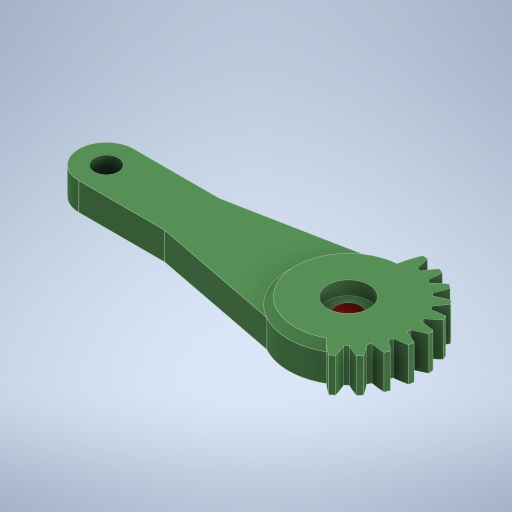
# Autodesk Inventor part: mechanism_1L
Saved by Autodesk Inventor 2023 (Build 270158000, 158)
## iProperties
Created: 2024-07-18
Part Number: mechanism_1L
Material: Generic
Document SubType Name: Modeling
Designer: Swoby
Density: 1 g/cm^3
Appearance: Default
Author: Swoby
Autodesk Inventor part; units mm, degrees
ref_plane "YZ Plane" through (0, 0, 0) normal (1, 0, 0) x (0, 1, 0)
ref_plane "XZ Plane" through (0, 0, 0) normal (0, 1, 0) x (-1, 0, 0)
ref_plane "XY Plane" through (0, 0, 0) normal (0, 0, 1) x (1, 0, 0)
sketch "Sketch1" plane through (0, 0, 0) normal (0, 1, 0) x (-1, 0, 0)
  circle A0 centre (0, 0) radius 1.75
  circle A1 centre (-35.232, 0) radius 1.75
  line L0 (0, 0) -> (-35.232, 0)
  line L1 (4, 0) -> (-39.232, 0) construction
  line L2 (0, -4) -> (-35.232, -4)
  line L3 (-35.232, 4) -> (-27.492, 4)
  arc A2 (0, -4) -> (0, 4) centre (0, 0) ccw
  arc A3 (-35.232, 4) -> (-35.232, -4) centre (-35.232, 0) ccw
  arc A4 (-26.5195, 0) -> (-27.492, 4) centre (-35.232, 0) ccw construction
  line L4 (-27.492, 4) -> (0, 4)
  arc A5 (-27.492, -4) -> (-26.5195, 0) centre (-35.232, 0) ccw construction
  arc A6 (-27.492, 4) -> (-27.492, -4) centre (-35.232, 0) ccw
  point P0 (-17.616, 0)
  dimension "d0" = 35.232
  dimension "d1" = 3.5
  dimension "d2" = 3.5
  dimension "d3" = 4
  dimension "d6" = 17.425
  constraints: 12 end point, 12 point on circle, 7 centre point, 6 tangent, 4 coincident, 4 point on line, 2 horizontal, 2 parallel, 1 midpoint
  measures "d0" distance of L0.end point (0, 0)
  measures "d1" diameter of A0
  measures "d2" diameter of A1
  measures "d3" radius of A2
  measures "d6" diameter of A4
extrude "Extrusion1" add sketch "Sketch1" along normal blind 4
sketch "Sketch2" plane through (0, 0, 0) normal (0, -1, 0) x (1, 0, 0)
  line L0 (27.492, -4) -> (0, -4) projected
  arc A0 (27.492, -4) -> (27.492, 4) centre (35.232, 0) ccw projected
  line L1 (0, 4) -> (27.492, 4) projected
  arc A1 (0, 4) -> (0, -4) centre (0, 0) ccw projected
  circle A2 centre (35.232, 0) radius 1.75 projected
  circle A3 centre (0, 0) radius 1.75 projected
  circle A4 centre (35.232, 0) radius 1.75 projected
  line L2 (35.232, 0) -> (35.232, -9.5201)
  line L3 (35.232, 0) -> (40.5265, 9.1703)
  arc A5 (35.232, -10.589) -> (40.5265, 9.1703) centre (35.232, 0) ccw
  line L4 (35.2321, 0.0005) -> (35.2321, 10.589) construction
  line L5 (35.2321, 0.0005) -> (40.5265, -9.1694) construction
  arc A6 (40.5265, -9.1694) -> (35.4759, -10.5852) centre (35.2321, 0.0005) ccw construction
  line L6 (35.2321, 0.0005) -> (42.6249, -4.6093) construction
  line L7 (35.2321, 0.0005) -> (42.7778, -4.3544) construction
  line L8 (35.2321, 0.0005) -> (42.4633, -4.8588) construction
  line L9 (35.2321, 0.0005) -> (43.506, -2.7279) construction
  line L10 (35.2321, 0.0005) -> (45.0385, -3.9936) construction
  line L11 (35.2321, 0.0005) -> (44.7425, -4.6546) construction
  arc A7 (45.0385, -3.9936) -> (43.506, -2.7279) centre (34.8965, -14.7131) ccw
  arc A8 (42.7778, -4.3544) -> (44.7425, -4.6546) centre (45.9843, 10.05) ccw
  arc A9 (44.7425, -4.6546) -> (45.0385, -3.9936) centre (35.2321, 0.0005) ccw
  arc A10 (42.4633, -4.8588) -> (42.7778, -4.3544) centre (35.2321, 0.0005) ccw
  line L12 (35.2321, 0.0005) -> (43.9353, -0.3948) construction
  line L13 (35.2321, 0.0005) -> (43.6728, -2.1574) construction
  line L14 (35.2321, 0.0005) -> (45.7524, -1.2001) construction
  line L15 (35.2321, 0.0005) -> (45.6457, -1.9165) construction
  arc A11 (43.6728, -2.1574) -> (43.9353, -0.3948) centre (35.2323, 0.0004) ccw construction
  arc A12 (43.506, -2.7279) -> (43.6728, -2.1574) centre (35.2323, 0.0004) ccw
  arc A13 (45.6457, -1.9165) -> (45.7524, -1.2001) centre (35.2321, 0.0005) ccw
  arc A14 (45.7524, -1.2001) -> (45.7767, 0.9637) centre (35.2321, 0.0005) ccw construction
  arc A15 (43.6728, -2.1574) -> (45.6457, -1.9165) centre (42.8748, 12.578) ccw
  arc A16 (45.7524, -1.2001) -> (43.9353, -0.3948) centre (38.8781, -14.2582) ccw
  line L16 (35.2321, 0.0005) -> (43.942, 0.1996) construction
  line L17 (35.2321, 0.0005) -> (45.7767, 0.9637) construction
  line L18 (35.2321, 0.0005) -> (45.6862, 1.6823) construction
  line L19 (35.2321, 0.0005) -> (43.7193, 1.9676) construction
  arc A17 (45.7767, 0.9637) -> (45.6862, 1.6823) centre (35.2321, 0.0005) ccw
  arc A18 (45.6862, 1.6823) -> (45.126, 3.7725) centre (35.2321, 0.0005) ccw construction
  arc A19 (43.942, 0.1996) -> (43.7193, 1.9676) centre (35.2323, 0.0004) ccw construction
  arc A20 (43.9353, -0.3948) -> (43.942, 0.1996) centre (35.2323, 0.0004) ccw
  arc A21 (43.7193, 1.9676) -> (43.5654, 2.5417) centre (35.2323, 0.0004) ccw
  arc A22 (43.942, 0.1996) -> (45.7767, 0.9637) centre (39.1986, 14.1734) ccw
  arc A23 (45.6862, 1.6823) -> (43.7193, 1.9676) centre (42.5894, -12.7461) ccw
  line L20 (35.2321, 0.0005) -> (43.5654, 2.5417) construction
  line L21 (35.2321, 0.0005) -> (45.126, 3.7725) construction
  line L22 (35.2321, 0.0005) -> (44.845, 4.4401) construction
  line L23 (35.2321, 0.0005) -> (42.874, 4.1841) construction
  line L24 (35.2321, 0.0005) -> (42.5709, 4.6955) construction
  line L25 (35.2321, 0.0005) -> (43.7417, 6.3016) construction
  line L26 (35.2321, 0.0005) -> (43.291, 6.8686) construction
  line L27 (35.2321, 0.0005) -> (41.4621, 6.0905) construction
  arc A24 (43.5654, 2.5417) -> (42.874, 4.1841) centre (35.2323, 0.0004) ccw construction
  arc A25 (42.5709, 4.6955) -> (41.4621, 6.0905) centre (35.2323, 0.0004) ccw construction
  arc A26 (42.874, 4.1841) -> (42.5709, 4.6955) centre (35.2323, 0.0004) ccw
  arc A27 (41.4621, 6.0905) -> (41.0323, 6.5011) centre (35.2323, 0.0004) ccw
  arc A28 (43.7417, 6.3016) -> (43.291, 6.8686) centre (35.2321, 0.0005) ccw
  arc A29 (43.291, 6.8686) -> (41.7264, 8.3636) centre (35.2321, 0.0005) ccw construction
  arc A30 (44.845, 4.4401) -> (43.7417, 6.3016) centre (35.2321, 0.0005) ccw construction
  arc A31 (45.126, 3.7725) -> (44.845, 4.4401) centre (35.2321, 0.0005) ccw
  arc A32 (43.291, 6.8686) -> (41.4621, 6.0905) centre (48.1409, -7.0686) ccw
  arc A33 (42.5709, 4.6955) -> (43.7417, 6.3016) centre (31.2583, 14.1714) ccw
  arc A34 (44.845, 4.4401) -> (42.874, 4.1841) centre (45.7553, -10.2888) ccw
  arc A35 (43.5654, 2.5417) -> (45.126, 3.7725) centre (35.2283, 14.718) ccw
  line L28 (35.2321, 0.0005) -> (41.0323, 6.5011) construction
  line L29 (35.2321, 0.0005) -> (41.7264, 8.3636) construction
  line L30 (35.2321, 0.0005) -> (41.1395, 8.788) construction
  line L31 (35.2321, 0.0005) -> (39.5882, 7.5452) construction
  arc A36 (41.7264, 8.3636) -> (41.1395, 8.788) centre (35.2321, 0.0005) ccw
  arc A37 (41.1395, 8.788) -> (35.2321, 10.589) centre (35.2321, 0.0005) ccw construction
  arc A38 (41.1395, 8.788) -> (39.5882, 7.5452) centre (49.5694, -3.3242) ccw
  arc A39 (41.0323, 6.5011) -> (41.7264, 8.3636) centre (27.5829, 12.5742) ccw
  line L32 (35.2321, 0.0005) -> (43.5975, -6.4908) construction
  line L33 (35.2321, 0.0005) -> (43.1341, -7.0475) construction
  line L34 (35.2321, 0.0005) -> (41.3233, -6.2284) construction
  line L35 (35.2321, 0.0005) -> (40.8844, -6.6293) construction
  line L36 (35.2321, 0.0005) -> (41.5362, -8.5068) construction
  line L37 (35.2321, 0.0005) -> (40.9399, -8.9179) construction
  line L38 (35.2321, 0.0005) -> (39.4172, -7.6407) construction
  line L39 (35.2321, 0.0005) -> (38.8864, -7.9082) construction
  line L40 (35.2321, 0.0005) -> (39.0076, -9.892) construction
  line L41 (35.2321, 0.0005) -> (38.3225, -10.127) construction
  line L42 (35.2321, 0.0005) -> (37.2007, -8.4863) construction
  line L43 (35.2321, 0.0005) -> (36.6174, -8.6008) construction
  line L44 (35.2321, 0.0005) -> (36.199, -10.5438) construction
  line L45 (35.2321, 0.0005) -> (35.4759, -10.5852) construction
  line L46 (35.2321, 0.0005) -> (34.8383, -8.7031) construction
  arc A40 (43.5975, -6.4908) -> (42.4633, -4.8588) centre (30.9397, -14.0771) ccw
  arc A41 (43.5975, -6.4908) -> (45.6457, -1.9165) centre (35.2321, 0.0005) ccw construction
  arc A42 (43.1341, -7.0475) -> (43.5975, -6.4908) centre (35.2321, 0.0005) ccw
  arc A43 (41.3233, -6.2284) -> (43.506, -2.7279) centre (35.2323, 0.0004) ccw construction
  arc A44 (40.8844, -6.6293) -> (41.3233, -6.2284) centre (35.2323, 0.0004) ccw
  arc A45 (40.9399, -8.9179) -> (41.5362, -8.5068) centre (35.2321, 0.0005) ccw
  arc A46 (41.5362, -8.5068) -> (43.1341, -7.0475) centre (35.2321, 0.0005) ccw construction
  arc A47 (38.3225, -10.127) -> (39.0076, -9.892) centre (35.2321, 0.0005) ccw
  arc A48 (39.0076, -9.892) -> (40.9399, -8.9179) centre (35.2321, 0.0005) ccw construction
  arc A49 (35.4759, -10.5852) -> (36.199, -10.5438) centre (35.2321, 0.0005) ccw
  arc A50 (36.199, -10.5438) -> (38.3225, -10.127) centre (35.2321, 0.0005) ccw construction
  arc A51 (38.8864, -7.9082) -> (39.4172, -7.6407) centre (35.2323, 0.0004) ccw
  arc A52 (39.4172, -7.6407) -> (40.8844, -6.6293) centre (35.2323, 0.0004) ccw construction
  arc A53 (37.2007, -8.4863) -> (38.8864, -7.9082) centre (35.2323, 0.0004) ccw construction
  arc A54 (36.6174, -8.6008) -> (37.2007, -8.4863) centre (35.2323, 0.0004) ccw
  arc A55 (41.3233, -6.2284) -> (43.1341, -7.0475) centre (48.2967, 6.777) ccw
  arc A56 (41.5362, -8.5068) -> (40.8844, -6.6293) centre (27.3013, -12.3973) ccw
  arc A57 (39.4172, -7.6407) -> (40.9399, -8.9179) centre (49.6404, 3.0014) ccw
  arc A58 (39.0076, -9.892) -> (38.8864, -7.9082) centre (24.2509, -9.7983) ccw
  arc A59 (37.2007, -8.4863) -> (38.3225, -10.127) centre (49.9158, -0.9967) ccw
  arc A60 (36.199, -10.5438) -> (36.6174, -8.6008) centre (22.0147, -6.4728) ccw
  arc A61 (34.8383, -8.7031) -> (35.4759, -10.5852) centre (49.1022, -4.92) ccw
  point P0 (37.8164, 8.3636)
  point P1 (39.5883, 7.5452)
  point P2 (42.7783, -4.3545)
  point P3 (42.4636, -4.8592)
  point P4 (41.3238, -6.2287)
  point P5 (40.8846, -6.6299)
  point P6 (39.4177, -7.6412)
  point P7 (38.8865, -7.909)
  point P8 (37.2012, -8.4871)
  point P9 (36.6173, -8.6017)
  point P10 (34.8385, -8.7036)
  point P11 (41.4621, 6.0905)
  point P12 (42.5709, 4.6955)
  point P13 (42.874, 4.1842)
  point P14 (43.5655, 2.5418)
  point P15 (43.7194, 1.9676)
  point P16 (43.9422, 0.1996)
  point P17 (43.9355, -0.3949)
  point P18 (43.6732, -2.1574)
  point P19 (43.5063, -2.7282)
  dimension "d9" = 150
  dimension "d7" = 150
  dimension "d8" = 10.589
  dimension "d10" = 10.5885
  dimension "d11" = 1.955
  dimension "d12" = 1.955
  dimension "d13" = 11.74
  dimension "d14" = 3.91
  dimension "d15" = 3.91
  dimension "d16" = 14.757
  dimension "d17" = 14.757
  dimension "d18" = 10.5885
  dimension "d19" = 3.91
  dimension "d20" = 3.91
  dimension "d21" = 3.91
  dimension "d22" = 11.74
  dimension "d23" = 14.757
  dimension "d24" = 14.757
  dimension "d25" = 3.91
  dimension "d26" = 3.91
  dimension "d27" = 3.91
  dimension "d28" = 11.74
  dimension "d29" = 14.757
  dimension "d30" = 14.757
  dimension "d31" = 3.91
  dimension "d32" = 3.91
  dimension "d33" = 3.91
  dimension "d34" = 11.74
  dimension "d35" = 3.91
  dimension "d36" = 3.91
  dimension "d37" = 11.74
  dimension "d38" = 3.91
  dimension "d39" = 14.757
  dimension "d40" = 14.757
  dimension "d41" = 14.757
  dimension "d42" = 14.757
  dimension "d43" = 3.91
  dimension "d44" = 3.91
  dimension "d45" = 11.74
  dimension "d46" = 3.91
  dimension "d47" = 14.757
  dimension "d48" = 14.757
  dimension "d49" = 3.91
  dimension "d50" = 3.91
  dimension "d51" = 11.74
  dimension "d52" = 3.91
  dimension "d53" = 3.91
  dimension "d54" = 3.91
  dimension "d55" = 11.74
  dimension "d56" = 3.91
  dimension "d57" = 3.91
  dimension "d58" = 3.91
  dimension "d59" = 11.74
  dimension "d60" = 3.91
  dimension "d61" = 3.91
  dimension "d62" = 3.91
  dimension "d63" = 11.74
  dimension "d64" = 14.757
  dimension "d65" = 14.757
  dimension "d66" = 14.757
  dimension "d67" = 14.757
  dimension "d68" = 14.757
  dimension "d69" = 14.757
  dimension "d70" = 14.757
  dimension "d71" = 14.757
  constraints: 167 point on circle, 56 centre point, 47 end point, 2 point on line, 1 coincident, 60 other
  measures "d7" angle of L2 L3
  measures "d8" radius of A5
  measures "d10" radius of A6
  measures "d11" angle of L6 L7
  measures "d12" angle of L8 L6
  measures "d13" angle of L7 L9
  measures "d14" angle of L10 L9
  measures "d15" angle of L7 L11
  measures "d16" radius of A7
  measures "d17" radius of A8
  measures "d18" radius of A9
  measures "d19" angle of L9 L13
  measures "d20" angle of L13 L15
  measures "d21" angle of L14 L12
  measures "d22" angle of L13 L12
  measures "d23" radius of A16
  measures "d24" radius of A15
  measures "d25" angle of L12 L16
  measures "d26" angle of L16 L17
  measures "d27" angle of L18 L19
  measures "d28" angle of L16 L19
  measures "d29" radius of A23
  measures "d30" radius of A22
  measures "d31" angle of L19 L20
  measures "d32" angle of L22 L23
  measures "d33" angle of L20 L21
  measures "d34" angle of L20 L23
  measures "d35" angle of L25 L24
  measures "d36" angle of L27 L26
  measures "d37" angle of L24 L27
  measures "d38" angle of L23 L24
  measures "d39" radius of A34
  measures "d40" radius of A35
  measures "d41" radius of A33
  measures "d42" radius of A32
  measures "d43" angle of L27 L28
  measures "d44" angle of L29 L28
  measures "d45" angle of L31 L28
  measures "d46" angle of L30 L31
  measures "d47" radius of A39
  measures "d48" radius of A38
  measures "d49" angle of L32 L8
  measures "d50" angle of L34 L33
  measures "d51" angle of L8 L34
  measures "d52" angle of L35 L34
  measures "d53" angle of L35 L36
  measures "d54" angle of L37 L38
  measures "d55" angle of L35 L38
  measures "d56" angle of L38 L39
  measures "d57" angle of L39 L40
  measures "d58" angle of L41 L42
  measures "d59" angle of L39 L42
  measures "d60" angle of L43 L42
  measures "d61" angle of L43 L44
  measures "d62" angle of L45 L46
  measures "d63" angle of L43 L46
  measures "d64" radius of A40
  measures "d65" radius of A55
  measures "d66" radius of A56
  measures "d67" radius of A57
  measures "d68" radius of A58
  measures "d69" radius of A59
  measures "d70" radius of A60
  measures "d71" radius of A61
extrude "Extrusion2" add sketch "Sketch2" against normal blind 4 contours A0 A60 A5 A61 | A38 A5 A39 A0 | A0 A58 A5 A59 | A32 A5 A33 A0 | A0 A56 A5 A57 | A34 A5 A35 A0 | A0 A40 A5 A55 | A23 A5 A22 A0 | A0 A7 A5 A8 | A16 A5 A15 A0
sketch "Sketch3" plane through (0, 4, 0) normal (0, 1, 0) x (1, 0, 0)
  line L0 (27.492, 4) -> (0, 4) projected
  arc A0 (0, 4) -> (0, -4) centre (0, 0) ccw projected
  line L1 (0, -4) -> (27.492, -4) projected
  arc A1 (27.492, -4) -> (39.5882, -7.5452) centre (35.232, 0) ccw projected
  arc A2 (39.5882, -7.5452) -> (41.1395, -8.788) centre (49.5694, 3.3242) ccw projected
  arc A3 (41.1395, -8.788) -> (41.7264, -8.3636) centre (35.2321, -0.0005) ccw projected
  arc A4 (41.7264, -8.3636) -> (41.0323, -6.5011) centre (27.5829, -12.5742) ccw projected
  arc A5 (41.0323, -6.5011) -> (41.4621, -6.0905) centre (35.232, 0) ccw projected
  arc A6 (41.4621, -6.0905) -> (43.291, -6.8686) centre (48.1409, 7.0686) ccw projected
  arc A7 (43.291, -6.8686) -> (43.7417, -6.3016) centre (35.2321, -0.0005) ccw projected
  arc A8 (43.7417, -6.3016) -> (42.5709, -4.6955) centre (31.2583, -14.1714) ccw projected
  arc A9 (42.5709, -4.6955) -> (42.874, -4.1842) centre (35.232, 0) ccw projected
  arc A10 (42.874, -4.1842) -> (44.845, -4.4401) centre (45.7553, 10.2888) ccw projected
  arc A11 (44.845, -4.4401) -> (45.126, -3.7725) centre (35.2321, -0.0005) ccw projected
  arc A12 (45.126, -3.7725) -> (43.5655, -2.5418) centre (35.2283, -14.718) ccw projected
  arc A13 (43.5655, -2.5418) -> (43.7194, -1.9676) centre (35.232, 0) ccw projected
  arc A14 (43.7194, -1.9676) -> (45.6862, -1.6823) centre (42.5894, 12.7461) ccw projected
  arc A15 (45.6862, -1.6823) -> (45.7767, -0.9637) centre (35.2321, -0.0005) ccw projected
  arc A16 (45.7767, -0.9637) -> (43.9422, -0.1996) centre (39.1986, -14.1734) ccw projected
  arc A17 (43.9422, -0.1996) -> (43.9355, 0.3949) centre (35.232, 0) ccw projected
  arc A18 (43.9355, 0.3949) -> (45.7524, 1.2001) centre (38.8781, 14.2582) ccw projected
  arc A19 (45.7524, 1.2001) -> (45.6457, 1.9165) centre (35.2321, -0.0005) ccw projected
  arc A20 (45.6457, 1.9165) -> (43.6732, 2.1574) centre (42.8748, -12.578) ccw projected
  arc A21 (43.6732, 2.1574) -> (43.5063, 2.7282) centre (35.232, 0) ccw projected
  arc A22 (43.5063, 2.7282) -> (45.0385, 3.9936) centre (34.8965, 14.7131) ccw projected
  arc A23 (45.0385, 3.9936) -> (44.7425, 4.6546) centre (35.2321, -0.0005) ccw projected
  arc A24 (44.7425, 4.6546) -> (42.7783, 4.3545) centre (45.9843, -10.05) ccw projected
  arc A25 (42.7783, 4.3545) -> (42.4636, 4.8592) centre (35.232, 0) ccw projected
  arc A26 (42.4636, 4.8592) -> (43.5975, 6.4908) centre (30.9397, 14.0771) ccw projected
  arc A27 (43.5975, 6.4908) -> (43.1341, 7.0475) centre (35.2321, -0.0005) ccw projected
  arc A28 (43.1341, 7.0475) -> (41.3238, 6.2287) centre (48.2967, -6.777) ccw projected
  arc A29 (41.3238, 6.2287) -> (40.8846, 6.6299) centre (35.232, 0) ccw projected
  arc A30 (40.8846, 6.6299) -> (41.5362, 8.5068) centre (27.3013, 12.3973) ccw projected
  arc A31 (41.5362, 8.5068) -> (40.9399, 8.9179) centre (35.2321, -0.0005) ccw projected
  arc A32 (40.9399, 8.9179) -> (39.4177, 7.6412) centre (49.6404, -3.0014) ccw projected
  arc A33 (39.4177, 7.6412) -> (38.8865, 7.909) centre (35.232, 0) ccw projected
  arc A34 (38.8865, 7.909) -> (39.0076, 9.892) centre (24.2509, 9.7983) ccw projected
  arc A35 (39.0076, 9.892) -> (38.3225, 10.127) centre (35.2321, -0.0005) ccw projected
  arc A36 (38.3225, 10.127) -> (37.2012, 8.4871) centre (49.9158, 0.9967) ccw projected
  arc A37 (37.2012, 8.4871) -> (36.6173, 8.6017) centre (35.232, 0) ccw projected
  arc A38 (36.6173, 8.6017) -> (36.199, 10.5438) centre (22.0147, 6.4728) ccw projected
  arc A39 (36.199, 10.5438) -> (35.4759, 10.5852) centre (35.2321, -0.0005) ccw projected
  arc A40 (35.4759, 10.5852) -> (34.8385, 8.7036) centre (49.1022, 4.92) ccw projected
  arc A41 (34.8385, 8.7036) -> (27.492, 4) centre (35.232, 0) ccw projected
  circle A42 centre (35.232, 0) radius 1.75 projected
  circle A43 centre (0, 0) radius 1.75 projected
  circle A44 centre (35.232, 0) radius 8.7125
  constraints: 1 coincident, 3 other
extrude "Extrusion3" add sketch "Sketch3" along normal blind 1 contours A41 A44 A37 A33 A29 A25 A21 A17 A13 A9 A5 A1 | A40 A39 A38 A44 | A44 A4 A3 A2 | A36 A35 A34 A44 | A44 A8 A7 A6 | A32 A31 A30 A44 | A44 A12 A11 A10 | A28 A27 A26 A44 | A44 A16 A15 A14 | A24 A23 A22 A44 | A20 A19 A18 A44
sketch "Sketch4" plane through (0, 5, 0) normal (0, 1, 0) x (1, 0, 0)
  circle A0 centre (35.232, 0) radius 1.75 projected
  circle A1 centre (35.232, 0) radius 3
  point P0 (0, 0)
  dimension "d77" = 6
  constraints: 1 centre point, 1 coincident
  measures "d77" diameter of A1
extrude "Extrusion4" cut sketch "Sketch4" against normal blind 2
chamfer "Chamfer1" distance 1 angle 45 1 edges at (26.8695, 5, 2.4445)
chamfer "Chamfer2" distance 15 distance2 5 1 edges at (27.492, 2, 4) measured on face at (26.992, 2, 4)
chamfer "Chamfer3" distance 15 distance2 5 1 edges at (27.492, 2, -4) measured on face at (26.992, 2, -4)
equation "\"d18\" = d10"
equation "\"d23\" = d16"
equation "\"d24\" = d17"
equation "\"d28\" = d22"
equation "\"d29\" = d17"
equation "\"d30\" = d24"
equation "\"d31\" = d27"
equation "\"d32\" = d31"
equation "\"d33\" = d31"
equation "\"d34\" = d22"
equation "\"d35\" = d33"
equation "\"d36\" = d35"
equation "\"d37\" = d34"
equation "\"d39\" = d29"
equation "\"d40\" = d39"
equation "\"d41\" = d40"
equation "\"d42\" = d40"
equation "\"d47\" = d41"
equation "\"d48\" = d41"
body "Solid1"
